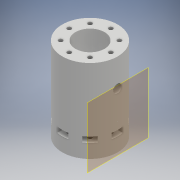
# Autodesk Inventor part: multiconnectorEndEffector
Saved by Autodesk Inventor 2017 (Build 210142000, 142)
## iProperties
Created: 2017-08-04
Part Number: multiconnectorEndEffector
Material: Generic
Document SubType Name: Sheet Metal
Designer: Bardo91
Density: 1 g/cm^3
Sheet Metal Rule: Default_mm
Appearance: Default
Author: Bardo91
Autodesk Inventor part; units mm, degrees
ref_plane "XZ Plane" through (0, 0, 0) normal (0, 1, 0) x (-1, 0, 0)
ref_plane "XY Plane" through (0, 0, 0) normal (0, 0, 1) x (1, 0, 0)
sketch "Sketch1" plane through (0, 0, 0) normal (0, 0, 1) x (1, 0, 0)
  circle A0 centre (0, 0) radius 10
  dimension "d0" = 20
  constraints: 1 centre point, 1 coincident
  measures "d0" diameter of A0
extrude "Extrusion1" add sketch "Sketch1" along normal blind 30
sketch "Sketch2" plane through (0, 0, 0) normal (0, 0, -1) x (-1, 0, 0)
  circle A0 centre (0, 0) radius 5
  dimension "d3" = 10
  constraints: 1 centre point, 1 coincident
  measures "d3" diameter of A0
extrude "Extrusion2" cut sketch "Sketch2" against normal blind 2
sketch "Sketch3" plane through (0, 0, 30) normal (0, 0, 1) x (1, 0, 0)
  line L0 (0, 0) -> (-7.5, 0)
  circle A0 centre (-7.5, 0) radius 0.75
  circle A1 centre (-5.3033, -5.3033) radius 0.75
  circle A2 centre (0, -7.5) radius 0.75
  circle A3 centre (5.3033, -5.3033) radius 0.75
  circle A4 centre (7.5, 0) radius 0.75
  circle A5 centre (5.3033, 5.3033) radius 0.75
  circle A6 centre (0, 7.5) radius 0.75
  circle A7 centre (-5.3033, 5.3033) radius 0.75
  dimension "d6" = 7.5
  dimension "d7" = 1.5
  dimension "d10" = 360
  constraints: 8 centre point, 2 end point, 1 coincident, 1 horizontal, 17 other
  measures "d6" distance of L0.start L0.end
  measures "d7" diameter of A0
extrude "Extrusion4" cut sketch "Sketch3" against normal up to surface (30 mm away)
ref_plane "Work Plane1" through (10, 0, 0) normal (1, 0, 0) x (0, 1, 0)
sketch "Sketch5" plane through (10, 0, 0) normal (1, 0, 0) x (0, 1, 0)
  line L0 (0, 0) -> (0, 5)
  line L1 (0, 5) -> (-2, 5)
  line L2 (-2, 5) -> (-2, 7)
  line L3 (-2, 7) -> (2, 7)
  line L4 (2, 7) -> (2, 5)
  line L5 (2, 5) -> (0, 5)
  dimension "d17" = 5
  dimension "d18" = 2
  dimension "d19" = 2
  dimension "d20" = 4
  constraints: 12 end point, 5 perpendicular, 1 point on line, 1 vertical
  measures "d17" distance of L0.start L0.end
  measures "d18" distance of L0.end L1.end
  measures "d19" distance of L1.end L2.end
  measures "d20" distance of L2.end L3.end
extrude "Extrusion5" cut sketch "Sketch5" against normal blind 5
pattern_circular "Circular Pattern1" count 8 over 360 about axis through (0, 0, 0) along (0, 0, 1) of "Extrusion5"
sketch "Sketch6" plane through (0, 0, 30) normal (0, 0, 1) x (1, 0, 0)
  circle A0 centre (0, 0) radius 5.25
  dimension "d26" = 10.5
  constraints: 1 centre point, 1 coincident
  measures "d26" diameter of A0
extrude "Extrusion6" cut sketch "Sketch6" against normal blind 15
sketch "Sketch7" plane through (10, 0, 0) normal (1, 0, 0) x (0, 1, 0)
  line L0 (10, 30) -> (-10, 30) projected
  line L1 (0, 30) -> (0, 20)
  circle A0 centre (0, 20) radius 1.5
  point P0 (0, 0)
  dimension "d29" = 10
  dimension "d30" = 3
  constraints: 2 end point, 1 centre point, 1 coincident, 1 midpoint, 1 vertical
  measures "d29" distance of L1.start L1.end
  measures "d30" diameter of A0
extrude "Extrusion7" cut sketch "Sketch7" against normal through all
equation "\"BendRadius\" = Thickness"
equation "\"BendReliefWidth\" = Thickness"
equation "\"BendReliefDepth\" = 0.5 * Thickness"
equation "\"CornerReliefSize\" = 4 * Thickness"
equation "\"MinimumRemnant\" = 2 * Thickness"
equation "\"TransitionRadius\" = BendRadius"
equation "\"JacobiRadiusSize\" = BendRadius"
equation "\"GapSize\" = Thickness"
equation "\"Thickness\" = 0.5"
body "Solid1"
